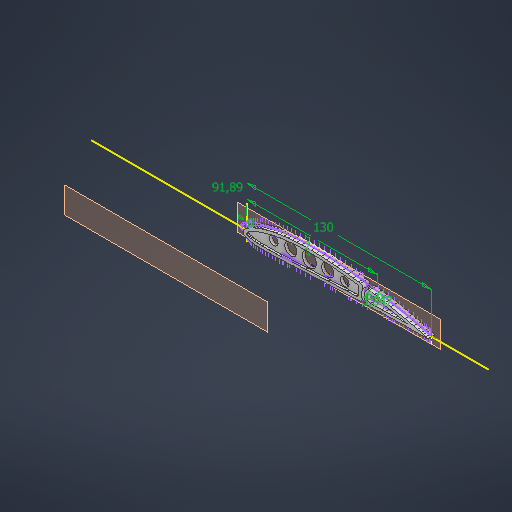
# Autodesk Inventor part: Profil NACA 4412 2
Saved by Autodesk Inventor 2026 (Build 300175050, 175E)
## iProperties
Created: 2026-02-20
Part Number: Profil NACA 4412 2
Material: Všeobecné
Document SubType Name: Modeling
Designer: marti
Density: 1 g/cm^3
Appearance: Výchozí
Author: marti
Autodesk Inventor part; units mm, degrees
ref_plane "YZ Plane" through (0, 0, 0) normal (1, 0, 0) x (0, 1, 0)
ref_plane "XZ Plane" through (0, 0, 0) normal (0, 1, 0) x (-1, 0, 0)
sketch "Náčrt1" plane through (0, 0, 0) normal (0, 0, 1) x (1, 0, 0)
  line L0 (0, 0.0009) -> (0.0949, -0.5809)
  line L1 (0.0949, -0.5809) -> (0.397, -1.1433)
  line L2 (0.397, -1.1433) -> (0.894, -1.646)
  line L3 (0.894, -1.646) -> (1.5811, -2.0907)
  line L4 (1.5811, -2.0907) -> (2.4535, -2.4793)
  line L5 (2.4535, -2.4793) -> (3.5069, -2.8138)
  line L6 (3.5069, -2.8138) -> (4.737, -3.0959)
  line L7 (4.737, -3.0959) -> (6.1391, -3.3275)
  line L8 (6.1391, -3.3275) -> (7.7086, -3.5107)
  line L9 (7.7086, -3.5107) -> (9.4408, -3.6478)
  line L10 (9.4408, -3.6478) -> (11.3308, -3.7411)
  line L11 (11.3308, -3.7411) -> (13.3737, -3.7933)
  line L12 (13.3737, -3.7933) -> (15.564, -3.7933)
  line L13 (15.564, -3.7933) -> (17.8973, -3.7933)
  line L14 (17.8973, -3.7933) -> (20.3676, -3.741)
  line L15 (20.3676, -3.741) -> (22.9712, -3.686)
  line L16 (22.9712, -3.686) -> (25.6984, -3.554)
  line L17 (25.6984, -3.554) -> (28.5465, -3.4161)
  line L18 (28.5465, -3.4161) -> (29.828, -3.3541)
  line L19 (29.828, -3.3541) -> (25.2693, -3.5754)
  line L20 (25.2693, -3.5754) -> (37.7531, -2.963)
  line L21 (37.7531, -2.963) -> (41.0259, -2.801)
  line L22 (41.0259, -2.801) -> (44.8539, -2.6115)
  line L23 (44.8539, -2.6115) -> (35.1018, -3.0226)
  line L24 (35.1018, -3.0226) -> (60.4375, -1.9699)
  line L25 (60.4375, -1.9699) -> (54.9288, -2.1938)
  line L26 (54.9288, -2.1938) -> (58.5738, -2.0455)
  line L27 (58.5738, -2.0455) -> (62.2711, -1.8951)
  line L28 (62.2711, -1.8951) -> (73.0297, -1.4573)
  line L29 (73.0297, -1.4573) -> (71.4832, -1.5215)
  line L30 (71.4832, -1.5215) -> (73.6, -1.435)
  line L31 (73.6, -1.435) -> (77.4223, -1.2826)
  line L32 (77.4223, -1.2826) -> (84.7627, -1.001)
  line L33 (87.2925, -0.9125) -> (102.9186, -0.3496)
  line L34 (102.9186, -0.3496) -> (98.1822, -0.524)
  line L35 (98.1822, -0.524) -> (96.4067, -0.572)
  line L36 (96.4067, -0.572) -> (100.0967, -0.4802)
  line L37 (100.0967, -0.4802) -> (103.7128, -0.3947)
  line L38 (103.7128, -0.3947) -> (107.2481, -0.3133)
  line L39 (107.2481, -0.3133) -> (110.6748, -0.2406)
  line L40 (110.6748, -0.2406) -> (113.9572, -0.1709)
  line L41 (113.9572, -0.1709) -> (117.1066, -0.2028)
  line L42 (117.1066, -0.2028) -> (120.0636, -0.1659)
  line L43 (120.0636, -0.1659) -> (122.7998, -0.136)
  line L44 (122.7998, -0.136) -> (127.2002, -0.0939)
  line L45 (127.2002, -0.0939) -> (127.3955, -0.0971)
  line L46 (127.3955, -0.0971) -> (129.0735, -0.125)
  line L47 (129.0735, -0.125) -> (129.9974, -0.1404)
  line L48 (129.9974, -0.1404) -> (129.9997, 0)
  line L49 (129.9997, 0) -> (128.6183, 0.5892)
  line L50 (128.6183, 0.5892) -> (126.8048, 1.0395)
  line L51 (126.8048, 1.0395) -> (125.2614, 1.446)
  line L52 (125.2614, 1.446) -> (122.7955, 2.0786)
  line L53 (122.7955, 2.0786) -> (120.0598, 2.7598)
  line L54 (120.0598, 2.7598) -> (117.1028, 3.472)
  line L55 (117.1028, 3.472) -> (113.9774, 4.2662)
  line L56 (113.9774, 4.2662) -> (110.6653, 4.9307)
  line L57 (110.6653, 4.9307) -> (107.233, 5.6192)
  line L58 (107.233, 5.6192) -> (103.7022, 6.3275)
  line L59 (103.7022, 6.3275) -> (100.087, 7.0517)
  line L60 (100.087, 7.0517) -> (96.4308, 7.7062)
  line L61 (96.4308, 7.7062) -> (92.6579, 8.3832)
  line L62 (92.6579, 8.3832) -> (87.9124, 9.1379)
  line L63 (82.4897, 9.9973) -> (81.2485, 10.1732)
  line L64 (81.2485, 10.1732) -> (77.4198, 10.673)
  line L65 (77.4198, 10.673) -> (73.598, 11.1279)
  line L66 (73.598, 11.1279) -> (69.7932, 11.5357)
  line L67 (69.7932, 11.5357) -> (66.0151, 11.8946)
  line L68 (66.0151, 11.8946) -> (62.2725, 12.2028)
  line L69 (62.2725, 12.2028) -> (58.5743, 12.4591)
  line L70 (58.5743, 12.4591) -> (54.9286, 12.6625)
  line L71 (54.9286, 12.6625) -> (51.3433, 12.8117)
  line L72 (51.3433, 12.8117) -> (47.8261, 12.889)
  line L73 (47.8261, 12.889) -> (44.3843, 12.8869)
  line L74 (44.3843, 12.8869) -> (41.025, 12.8075)
  line L75 (41.025, 12.8075) -> (37.755, 12.6532)
  line L76 (37.755, 12.6532) -> (34.5809, 12.4269)
  line L77 (34.5809, 12.4269) -> (31.509, 12.1323)
  line L78 (31.509, 12.1323) -> (28.5458, 11.773)
  line L79 (28.5458, 11.773) -> (25.6971, 11.3534)
  line L80 (25.6971, 11.3534) -> (22.969, 10.8781)
  line L81 (22.969, 10.8781) -> (20.367, 10.352)
  line L82 (20.367, 10.352) -> (17.8969, 9.7802)
  line L83 (17.8969, 9.7802) -> (15.564, 9.1684)
  line L84 (15.564, 9.1684) -> (13.3737, 8.522)
  line L85 (13.3737, 8.522) -> (11.3313, 7.8468)
  line L86 (11.3313, 7.8468) -> (9.4417, 7.1485)
  line L87 (9.4417, 7.1485) -> (7.7101, 6.433)
  line L88 (7.7101, 6.433) -> (6.1413, 5.7058)
  line L89 (6.1413, 5.7058) -> (4.74, 4.9723)
  line L90 (4.74, 4.9723) -> (3.5111, 4.2378)
  line L91 (3.5111, 4.2378) -> (2.4591, 3.5071)
  line L92 (2.4591, 3.5071) -> (1.5886, 2.7846)
  line L93 (1.5886, 2.7846) -> (0.904, 2.0741)
  line L94 (0.904, 2.0741) -> (0.4097, 1.379)
  line L95 (0.4097, 1.379) -> (0.1113, 0.7047)
  line L96 (0.1113, 0.7047) -> (0, 0.0009)
  line L97 (41.0958, 10.8086) -> (44.4086, 10.8869)
  line L98 (44.4086, 10.8869) -> (47.8048, 10.889)
  line L99 (47.8048, 10.889) -> (51.2798, 10.8126)
  line L100 (51.2798, 10.8126) -> (54.8313, 10.6648)
  line L101 (54.8313, 10.6648) -> (58.4495, 10.4629)
  line L102 (58.4495, 10.4629) -> (62.1213, 10.2085)
  line L103 (62.1213, 10.2085) -> (65.8384, 9.9023)
  line L104 (65.8384, 9.9023) -> (69.5921, 9.5458)
  line L105 (69.5921, 9.5458) -> (73.3732, 9.1405)
  line L106 (73.3732, 9.1405) -> (77.1721, 8.6884)
  line L107 (77.1721, 8.6884) -> (80.9788, 8.1915)
  line L108 (80.9788, 8.1915) -> (82.1224, 8.0294)
  line L109 (92.3241, 6.4112) -> (96.0779, 5.7375)
  line L110 (96.0779, 5.7375) -> (99.7143, 5.0866)
  line L111 (99.7143, 5.0866) -> (103.3091, 4.3665)
  line L112 (103.3091, 4.3665) -> (106.8235, 3.6615)
  line L113 (106.8235, 3.6615) -> (110.2382, 2.9765)
  line L114 (110.2382, 2.9765) -> (113.5341, 2.3153)
  line L115 (113.5341, 2.3153) -> (115.5088, 1.8135)
  line L116 (115.5088, 1.8135) -> (113.9461, 1.8293)
  line L117 (113.9461, 1.8293) -> (110.6323, 1.759)
  line L118 (110.6323, 1.759) -> (107.2038, 1.6862)
  line L119 (107.2038, 1.6862) -> (103.6661, 1.6047)
  line L120 (103.6661, 1.6047) -> (100.0482, 1.5192)
  line L121 (100.0482, 1.5192) -> (96.3548, 1.4273)
  line L122 (96.3548, 1.4273) -> (98.1184, 1.475)
  line L123 (98.1184, 1.475) -> (102.8646, 1.6498)
  line L124 (102.8646, 1.6498) -> (88.1854, 1.1209)
  line L125 (81.6875, 0.8825) -> (77.3447, 0.7159)
  line L126 (77.3447, 0.7159) -> (73.5193, 0.5634)
  line L127 (73.5193, 0.5634) -> (71.4009, 0.4768)
  line L128 (71.4009, 0.4768) -> (72.9476, 0.541)
  line L129 (72.9476, 0.541) -> (62.1898, 0.1033)
  line L130 (62.1898, 0.1033) -> (58.4925, -0.0472)
  line L131 (58.4925, -0.0472) -> (54.8476, -0.1955)
  line L132 (54.8476, -0.1955) -> (60.3554, 0.0284)
  line L133 (60.3554, 0.0284) -> (35.0182, -1.0243)
  line L134 (35.0182, -1.0243) -> (44.7624, -0.6136)
  line L135 (44.7624, -0.6136) -> (40.9263, -0.8035)
  line L136 (40.9263, -0.8035) -> (37.6546, -0.9654)
  line L137 (37.6546, -0.9654) -> (25.1718, -1.5778)
  line L138 (25.1718, -1.5778) -> (29.7312, -1.3564)
  line L139 (29.7312, -1.3564) -> (28.4563, -1.4181)
  line L140 (28.4563, -1.4181) -> (25.6082, -1.556)
  line L141 (25.6082, -1.556) -> (22.9017, -1.687)
  line L142 (22.9017, -1.687) -> (20.3188, -1.7416)
  line L143 (20.3188, -1.7416) -> (17.8761, -1.7933)
  line L144 (17.8761, -1.7933) -> (15.564, -1.7933)
  line L145 (15.564, -1.7933) -> (13.3992, -1.7933)
  line L146 (13.3992, -1.7933) -> (11.4056, -1.7424)
  line L147 (11.4056, -1.7424) -> (9.569, -1.6517)
  line L148 (9.569, -1.6517) -> (7.9035, -1.5199)
  line L149 (7.9035, -1.5199) -> (6.4182, -1.3465)
  line L150 (6.4182, -1.3465) -> (5.1239, -1.1327)
  line L151 (5.1239, -1.1327) -> (4.034, -0.8827)
  line L152 (4.034, -0.8827) -> (3.1652, -0.6069)
  line L153 (3.1652, -0.6069) -> (2.5371, -0.3271)
  line L154 (2.5371, -0.3271) -> (2.1633, -0.0851)
  line L155 (2.1633, -0.0851) -> (2.0322, 0.0474)
  line L156 (2.0322, 0.0474) -> (2.046, 0.1343)
  line L157 (2.046, 0.1343) -> (2.1568, 0.3847)
  line L158 (2.1568, 0.3847) -> (2.4476, 0.7937)
  line L159 (2.4476, 0.7937) -> (2.9515, 1.3167)
  line L160 (2.9515, 1.3167) -> (3.6705, 1.9134)
  line L161 (3.6705, 1.9134) -> (4.5959, 2.5562)
  line L162 (4.5959, 2.5562) -> (5.7176, 3.2266)
  line L163 (5.7176, 3.2266) -> (7.0261, 3.9115)
  line L164 (7.0261, 3.9115) -> (8.5129, 4.6007)
  line L165 (8.5129, 4.6007) -> (10.1705, 5.2857)
  line L166 (10.1705, 5.2857) -> (11.992, 5.9587)
  line L167 (11.992, 5.9587) -> (13.9708, 6.6129)
  line L168 (13.9708, 6.6129) -> (16.1009, 7.2416)
  line L169 (16.1009, 7.2416) -> (18.3762, 7.8383)
  line L170 (18.3762, 7.8383) -> (20.7908, 8.3972)
  line L171 (20.7908, 8.3972) -> (23.3389, 8.9124)
  line L172 (23.3389, 8.9124) -> (26.0146, 9.3786)
  line L173 (26.0146, 9.3786) -> (28.8119, 9.7907)
  line L174 (28.8119, 9.7907) -> (31.7249, 10.1438)
  line L175 (31.7249, 10.1438) -> (34.7474, 10.4337)
  line L176 (34.7474, 10.4337) -> (37.8732, 10.6565)
  line L177 (37.8732, 10.6565) -> (41.0958, 10.8086)
  line L178 (0, 16.2255) -> (0, -7.1297) projected
  line L179 (-109.522, 0) -> (169.92, 0) projected
  arc A0 (85.4115, 9.5353) -> (84.7627, -1.001) centre (91.8618, 3.85) ccw
  arc A1 (87.9203, 9.1438) -> (87.2925, -0.9125) centre (91.8618, 3.85) ccw
  line L180 (85.4115, 9.5353) -> (82.4897, 9.9973)
  arc A2 (92.7028, 8.3752) -> (92.6128, 8.3904) centre (91.8903, 3.8474) ccw
  line L181 (88.551, 7.0112) -> (92.3241, 6.4112)
  arc A3 (82.1224, 8.0294) -> (81.6875, 0.8825) centre (91.8618, 3.85) ccw
  arc A4 (88.551, 7.0112) -> (88.1854, 1.1209) centre (91.8903, 3.8474) ccw
  point P0 (0, 0)
  point P1 (0.0092, 0.0443)
  point P2 (80.0237, 10.3925)
  point P3 (81.2485, -1.1461)
  point P4 (85.0783, -0.9923)
  point P5 (0, -1.8302)
  point P6 (0, -1.8314)
  point P7 (72.2186, -1.4898)
  point P8 (-4.2032, 0)
  point P9 (0, 0.1702)
  point P10 (129.7617, -0.163)
  point P11 (0, 11.0071)
  point P12 (0, -1.8299)
  point P13 (41.3587, -2.7449)
  point P14 (41.277, -0.7466)
  point P15 (0, 8.9957)
  point P16 (0, 0.1718)
  point P17 (0, 0.1714)
  point P18 (-69.6017, 0)
  point P19 (72.1378, 0.5085)
  point P20 (26.1583, -1.5294)
  point P21 (59.6518, 0)
  point P22 (2.0791, 0)
  point P23 (26.2556, -3.527)
  point P24 (44.1123, -2.6482)
  point P25 (44.0214, -0.6503)
  point P26 (59.6564, 0)
  point P27 (97.4348, 1.4542)
  point P28 (97.4969, -0.5449)
  point P29 (97.7601, -0.5354)
  point P30 (87.9124, 9.1379)
  point P31 (97.6955, 1.4636)
  point P32 (59.6716, 0)
  dimension "d0" = 2
  dimension "d1" = 0
  dimension "d10" = 129.9997
  dimension "d12" = 3.8474
  dimension "d13" = 91.8903
  dimension "d17" = 6.6
  constraints: 360 end point, 12 collinear, 11 point on circle, 5 centre point, 3 coincident, 3 point on line, 2 parallel, 2 perpendicular, 2 tangent, 1 horizontal, 75 other
  measures "d0" distance between parallel lines of L74 L97
  measures "d1" distance from line of L178 point (0, 0.001)
  measures "d10" distance of L48.end point (0, 0.001)
  measures "d12" distance from line of L179 A2.centre
  measures "d13" distance from line of L178 A2.centre
  measures "d17" radius of A1
ref_plane "Pracovní rovina1" through (0, 0, 50) normal (0, 0, 1) x (1, 0, 0)
sketch "Náčrt2" plane through (0.1197, -0.0139, 50) normal (0, 0, 1) x (1, 0, 0)
  line L0 (-71.7303, -0.321) -> (-71.6354, -0.9019)
  line L1 (-71.6354, -0.9019) -> (-71.3333, -1.4643)
  line L2 (-71.3333, -1.4643) -> (-70.8362, -1.967)
  line L3 (-70.8362, -1.967) -> (-70.1492, -2.4117)
  line L4 (-70.1492, -2.4117) -> (-69.2768, -2.8003)
  line L5 (-69.2768, -2.8003) -> (-68.2233, -3.1347)
  line L6 (-68.2233, -3.1347) -> (-66.9933, -3.4168)
  line L7 (-66.9933, -3.4168) -> (-65.5912, -3.6485)
  line L8 (-65.5912, -3.6485) -> (-64.0217, -3.8317)
  line L9 (-64.0217, -3.8317) -> (-62.2895, -3.9688)
  line L10 (-62.2895, -3.9688) -> (-60.3995, -4.0621)
  line L11 (-60.3995, -4.0621) -> (-58.3565, -4.1142)
  line L12 (-58.3565, -4.1142) -> (-56.1662, -4.1142)
  line L13 (-56.1662, -4.1142) -> (-53.833, -4.1142)
  line L14 (-53.833, -4.1142) -> (-51.3627, -4.062)
  line L15 (-51.3627, -4.062) -> (-48.7592, -4.0069)
  line L16 (-48.7592, -4.0069) -> (-46.0319, -3.8749)
  line L17 (-46.0319, -3.8749) -> (-43.1838, -3.7371)
  line L18 (-43.1838, -3.7371) -> (-40.2179, -3.5936)
  line L19 (-40.2179, -3.5936) -> (-37.15, -3.4367)
  line L20 (-37.15, -3.4367) -> (-33.9745, -3.2772)
  line L21 (-33.9745, -3.2772) -> (-30.7049, -3.1104)
  line L22 (-30.7049, -3.1104) -> (-27.346, -2.9391)
  line L23 (-27.346, -2.9391) -> (-23.9054, -2.7954)
  line L24 (-23.9054, -2.7954) -> (-23.4055, -2.7752)
  line L25 (-23.4055, -2.7752) -> (-16.802, -2.5148)
  line L26 (-16.802, -2.5148) -> (-13.1565, -2.3665)
  line L27 (-13.1565, -2.3665) -> (-9.459, -2.216)
  line L28 (-9.459, -2.216) -> (1.2996, -1.7761)
  line L29 (1.2996, -1.7761) -> (-1.939, -1.9065)
  line L30 (-1.939, -1.9065) -> (1.8675, -1.757)
  line L31 (1.8675, -1.757) -> (5.6913, -1.6068)
  line L32 (5.6913, -1.6068) -> (13.346, -1.3203)
  line L33 (13.346, -1.3203) -> (17.1555, -1.1884)
  line L34 (17.1555, -1.1884) -> (20.9379, -1.0676)
  line L35 (20.9379, -1.0676) -> (24.6804, -0.9571)
  line L36 (24.6804, -0.9571) -> (28.3686, -0.8572)
  line L37 (28.3686, -0.8572) -> (31.9862, -0.7683)
  line L38 (31.9862, -0.7683) -> (35.5166, -0.6903)
  line L39 (35.5166, -0.6903) -> (38.9405, -0.6229)
  line L40 (38.9405, -0.6229) -> (42.2338, -0.5655)
  line L41 (42.2338, -0.5655) -> (45.3763, -0.5685)
  line L42 (45.3763, -0.5685) -> (48.3339, -0.5316)
  line L43 (48.3339, -0.5316) -> (51.07, -0.5017)
  line L44 (51.07, -0.5017) -> (53.5363, -0.4781)
  line L45 (53.5363, -0.4781) -> (55.6645, -0.46)
  line L46 (55.6645, -0.46) -> (57.343, -0.4458)
  line L47 (57.343, -0.4458) -> (58.272, -0.4379)
  line L48 (58.272, -0.4379) -> (58.2695, -0.1446)
  line L49 (58.2695, -0.1446) -> (57.3365, 0.1109)
  line L50 (57.3365, 0.1109) -> (55.6584, 0.5623)
  line L51 (55.6584, 0.5623) -> (53.5305, 1.1227)
  line L52 (53.5305, 1.1227) -> (51.0647, 1.7553)
  line L53 (51.0647, 1.7553) -> (48.329, 2.4365)
  line L54 (48.329, 2.4365) -> (45.372, 3.1487)
  line L55 (45.372, 3.1487) -> (42.2483, 3.9465)
  line L56 (42.2483, 3.9465) -> (38.9352, 4.6104)
  line L57 (38.9352, 4.6104) -> (35.5028, 5.2982)
  line L58 (35.5028, 5.2982) -> (31.9708, 6.006)
  line L59 (31.9708, 6.006) -> (28.356, 6.7272)
  line L60 (28.356, 6.7272) -> (24.6665, 7.3905)
  line L61 (24.6665, 7.3905) -> (20.9275, 8.0618)
  line L62 (20.9275, 8.0618) -> (17.1433, 8.6633)
  line L63 (17.1433, 8.6633) -> (10.7595, 9.6764)
  line L64 (10.7595, 9.6764) -> (9.5183, 9.8523)
  line L65 (9.5183, 9.8523) -> (5.6895, 10.352)
  line L66 (5.6895, 10.352) -> (1.8677, 10.8069)
  line L67 (1.8677, 10.8069) -> (-1.937, 11.2148)
  line L68 (-1.937, 11.2148) -> (-5.7152, 11.5736)
  line L69 (-5.7152, 11.5736) -> (-9.4577, 11.8818)
  line L70 (-9.4577, 11.8818) -> (-13.156, 12.1381)
  line L71 (-13.156, 12.1381) -> (-16.8017, 12.3415)
  line L72 (-16.8017, 12.3415) -> (-20.3869, 12.4907)
  line L73 (-20.3869, 12.4907) -> (-23.9041, 12.568)
  line L74 (-23.9041, 12.568) -> (-27.3459, 12.5659)
  line L75 (-27.3459, 12.5659) -> (-30.7053, 12.4865)
  line L76 (-30.7053, 12.4865) -> (-33.9753, 12.3322)
  line L77 (-33.9753, 12.3322) -> (-37.1494, 12.106)
  line L78 (-37.1494, 12.106) -> (-40.2212, 11.8113)
  line L79 (-40.2212, 11.8113) -> (-43.1845, 11.4521)
  line L80 (-43.1845, 11.4521) -> (-46.0331, 11.0325)
  line L81 (-46.0331, 11.0325) -> (-48.7613, 10.5571)
  line L82 (-48.7613, 10.5571) -> (-51.3633, 10.031)
  line L83 (-51.3633, 10.031) -> (-53.8334, 9.4593)
  line L84 (-53.8334, 9.4593) -> (-56.1663, 8.8474)
  line L85 (-56.1663, 8.8474) -> (-58.3565, 8.201)
  line L86 (-58.3565, 8.201) -> (-60.399, 7.5258)
  line L87 (-60.399, 7.5258) -> (-62.2885, 6.8276)
  line L88 (-62.2885, 6.8276) -> (-64.0202, 6.112)
  line L89 (-64.0202, 6.112) -> (-65.589, 5.3848)
  line L90 (-65.589, 5.3848) -> (-66.9902, 4.6513)
  line L91 (-66.9902, 4.6513) -> (-68.2191, 3.9168)
  line L92 (-68.2191, 3.9168) -> (-69.2711, 3.1861)
  line L93 (-69.2711, 3.1861) -> (-70.1417, 2.4636)
  line L94 (-70.1417, 2.4636) -> (-70.8263, 1.7531)
  line L95 (-70.8263, 1.7531) -> (-71.3206, 1.058)
  line L96 (-71.3206, 1.058) -> (-71.6181, 0.3856)
  line L97 (-71.6181, 0.3856) -> (-71.7303, -0.321)
  line L98 (-30.6345, 10.4876) -> (-27.3217, 10.566)
  line L99 (-27.3217, 10.566) -> (-23.9255, 10.568)
  line L100 (-23.9255, 10.568) -> (-20.4505, 10.4916)
  line L101 (-20.4505, 10.4916) -> (-16.899, 10.3438)
  line L102 (-16.899, 10.3438) -> (-13.2808, 10.142)
  line L103 (-13.2808, 10.142) -> (-9.6089, 9.8875)
  line L104 (-9.6089, 9.8875) -> (-5.8918, 9.5814)
  line L105 (-5.8918, 9.5814) -> (-2.1382, 9.2249)
  line L106 (-2.1382, 9.2249) -> (1.6429, 8.8196)
  line L107 (1.6429, 8.8196) -> (5.4419, 8.3674)
  line L108 (5.4419, 8.3674) -> (9.2485, 7.8705)
  line L109 (9.2485, 7.8705) -> (10.4624, 7.6985)
  line L110 (10.4624, 7.6985) -> (16.8296, 6.6881)
  line L111 (16.8296, 6.6881) -> (20.5938, 6.0898)
  line L112 (20.5938, 6.0898) -> (24.3128, 5.422)
  line L113 (24.3128, 5.422) -> (27.9834, 4.7621)
  line L114 (27.9834, 4.7621) -> (31.5786, 4.0448)
  line L115 (31.5786, 4.0448) -> (35.0933, 3.3405)
  line L116 (35.0933, 3.3405) -> (38.508, 2.6563)
  line L117 (38.508, 2.6563) -> (41.8041, 1.9958)
  line L118 (41.8041, 1.9958) -> (44.0083, 1.4328)
  line L119 (44.0083, 1.4328) -> (42.2173, 1.4345)
  line L120 (42.2173, 1.4345) -> (38.9034, 1.3767)
  line L121 (38.9034, 1.3767) -> (35.4748, 1.3092)
  line L122 (35.4748, 1.3092) -> (31.9395, 1.2311)
  line L123 (31.9395, 1.2311) -> (28.3169, 1.1421)
  line L124 (28.3169, 1.1421) -> (24.6238, 1.0421)
  line L125 (24.6238, 1.0421) -> (20.8764, 0.9314)
  line L126 (20.8764, 0.9314) -> (17.089, 0.8105)
  line L127 (17.089, 0.8105) -> (13.274, 0.6784)
  line L128 (13.274, 0.6784) -> (5.6146, 0.3917)
  line L129 (5.6146, 0.3917) -> (1.789, 0.2415)
  line L130 (1.789, 0.2415) -> (-2.0185, 0.0919)
  line L131 (-2.0185, 0.0919) -> (1.2185, 0.2222)
  line L132 (1.2185, 0.2222) -> (-9.5405, -0.2177)
  line L133 (-9.5405, -0.2177) -> (-13.2378, -0.3681)
  line L134 (-13.2378, -0.3681) -> (-16.8821, -0.5164)
  line L135 (-16.8821, -0.5164) -> (-23.4852, -0.7768)
  line L136 (-23.4852, -0.7768) -> (-23.9874, -0.797)
  line L137 (-23.9874, -0.797) -> (-27.4387, -0.9412)
  line L138 (-27.4387, -0.9412) -> (-30.8046, -1.1129)
  line L139 (-30.8046, -1.1129) -> (-34.0757, -1.2797)
  line L140 (-34.0757, -1.2797) -> (-37.2512, -1.4393)
  line L141 (-37.2512, -1.4393) -> (-40.3173, -1.596)
  line L142 (-40.3173, -1.596) -> (-43.274, -1.7391)
  line L143 (-43.274, -1.7391) -> (-46.122, -1.877)
  line L144 (-46.122, -1.877) -> (-48.8287, -2.008)
  line L145 (-48.8287, -2.008) -> (-51.4115, -2.0626)
  line L146 (-51.4115, -2.0626) -> (-53.8541, -2.1142)
  line L147 (-53.8541, -2.1142) -> (-56.1662, -2.1142)
  line L148 (-56.1662, -2.1142) -> (-58.331, -2.1142)
  line L149 (-58.331, -2.1142) -> (-60.3246, -2.0633)
  line L150 (-60.3246, -2.0633) -> (-62.1613, -1.9727)
  line L151 (-62.1613, -1.9727) -> (-63.8267, -1.8409)
  line L152 (-63.8267, -1.8409) -> (-65.3121, -1.6675)
  line L153 (-65.3121, -1.6675) -> (-66.6064, -1.4537)
  line L154 (-66.6064, -1.4537) -> (-67.6963, -1.2037)
  line L155 (-67.6963, -1.2037) -> (-68.565, -0.9279)
  line L156 (-68.565, -0.9279) -> (-69.1931, -0.6481)
  line L157 (-69.1931, -0.6481) -> (-69.5669, -0.4061)
  line L158 (-69.5669, -0.4061) -> (-69.6978, -0.2738)
  line L159 (-69.6978, -0.2738) -> (-69.6837, -0.1853)
  line L160 (-69.6837, -0.1853) -> (-69.5735, 0.0638)
  line L161 (-69.5735, 0.0638) -> (-69.2827, 0.4727)
  line L162 (-69.2827, 0.4727) -> (-68.7787, 0.9957)
  line L163 (-68.7787, 0.9957) -> (-68.0598, 1.5924)
  line L164 (-68.0598, 1.5924) -> (-67.1344, 2.2352)
  line L165 (-67.1344, 2.2352) -> (-66.0127, 2.9056)
  line L166 (-66.0127, 2.9056) -> (-64.7042, 3.5905)
  line L167 (-64.7042, 3.5905) -> (-63.2174, 4.2797)
  line L168 (-63.2174, 4.2797) -> (-61.5597, 4.9647)
  line L169 (-61.5597, 4.9647) -> (-59.7383, 5.6378)
  line L170 (-59.7383, 5.6378) -> (-57.7594, 6.292)
  line L171 (-57.7594, 6.292) -> (-55.6294, 6.9206)
  line L172 (-55.6294, 6.9206) -> (-53.3541, 7.5173)
  line L173 (-53.3541, 7.5173) -> (-50.9395, 8.0762)
  line L174 (-50.9395, 8.0762) -> (-48.3914, 8.5915)
  line L175 (-48.3914, 8.5915) -> (-45.7157, 9.0576)
  line L176 (-45.7157, 9.0576) -> (-42.9184, 9.4697)
  line L177 (-42.9184, 9.4697) -> (-40.0053, 9.8229)
  line L178 (-40.0053, 9.8229) -> (-36.9828, 10.1128)
  line L179 (-36.9828, 10.1128) -> (-33.857, 10.3355)
  line L180 (-33.857, 10.3355) -> (-30.6345, 10.4876)
  line L181 (0, 15.9045) -> (0, -7.4507)
  line L182 (-97.7307, 0) -> (84.2724, 0)
  point P0 (0, 0)
  point P1 (-71.7211, -0.2767)
  point P2 (9.5183, -1.467)
  point P3 (0, -1.8293)
  point P4 (0, -1.8303)
  point P5 (-0.6652, -1.8565)
  point P6 (-4.2164, 0)
  point P7 (0, 0.1712)
  dimension "d6" = 2
  dimension "d5" = 71.7303
  constraints: 366 end point, 12 collinear, 3 perpendicular, 2 parallel, 1 coincident, 1 horizontal, 82 other
  measures "d6" distance between parallel lines of L75 L98
  measures "d5" distance from line of L181 point (-71.73, -0.321)
extrude "Vysunutí2" [suppressed]
ref_plane "Pracovní rovina3" through (0, 0, 0) normal (0, 0, 1) x (1, 0, 0)
sketch "Náčrt3" plane through (0, 0, 0) normal (0, 0, 1) x (1, 0, 0)
  arc A0 (83.961, 7.2422) -> (82.4897, 9.9973) centre (82.1232, 8.0312) ccw projected
  line L0 (82.4897, 9.9973) -> (81.2485, 10.1732) projected
  line L1 (81.2485, 10.1732) -> (77.4198, 10.673) projected
  line L2 (77.4198, 10.673) -> (73.598, 11.1279) projected
  line L3 (73.598, 11.1279) -> (69.7932, 11.5357) projected
  line L4 (69.7932, 11.5357) -> (66.0151, 11.8946) projected
  line L5 (66.0151, 11.8946) -> (62.2725, 12.2028) projected
  line L6 (62.2725, 12.2028) -> (58.5743, 12.4591) projected
  line L7 (58.5743, 12.4591) -> (54.9286, 12.6625) projected
  line L8 (54.9286, 12.6625) -> (51.3433, 12.8117) projected
  line L9 (51.3433, 12.8117) -> (47.8261, 12.889) projected
  line L10 (47.8261, 12.889) -> (44.3843, 12.8869) projected
  line L11 (44.3843, 12.8869) -> (41.025, 12.8075) projected
  line L12 (41.025, 12.8075) -> (37.755, 12.6532) projected
  line L13 (37.755, 12.6532) -> (34.5809, 12.4269) projected
  line L14 (34.5809, 12.4269) -> (31.509, 12.1323) projected
  line L15 (31.509, 12.1323) -> (28.5458, 11.773) projected
  line L16 (28.5458, 11.773) -> (25.6971, 11.3534) projected
  line L17 (25.6971, 11.3534) -> (22.969, 10.8781) projected
  line L18 (22.969, 10.8781) -> (20.367, 10.352) projected
  line L19 (20.367, 10.352) -> (17.8969, 9.7802) projected
  line L20 (17.8969, 9.7802) -> (15.564, 9.1684) projected
  line L21 (15.564, 9.1684) -> (13.3737, 8.522) projected
  line L22 (13.3737, 8.522) -> (11.3313, 7.8468) projected
  line L23 (11.3313, 7.8468) -> (9.4417, 7.1485) projected
  line L24 (9.4417, 7.1485) -> (7.7101, 6.433) projected
  line L25 (7.7101, 6.433) -> (6.1413, 5.7058) projected
  line L26 (6.1413, 5.7058) -> (4.74, 4.9723) projected
  line L27 (4.74, 4.9723) -> (3.5111, 4.2378) projected
  line L28 (3.5111, 4.2378) -> (2.4591, 3.5071) projected
  line L29 (2.4591, 3.5071) -> (1.5886, 2.7846) projected
  line L30 (1.5886, 2.7846) -> (0.904, 2.0741) projected
  line L31 (0.904, 2.0741) -> (0.4097, 1.379) projected
  line L32 (0.4097, 1.379) -> (0.1113, 0.7047) projected
  line L33 (0.1113, 0.7047) -> (0, 0.0009) projected
  line L34 (0, 0.0009) -> (0.0949, -0.5809) projected
  line L35 (0.0949, -0.5809) -> (0.397, -1.1433) projected
  line L36 (0.397, -1.1433) -> (0.894, -1.646) projected
  line L37 (0.894, -1.646) -> (1.5811, -2.0907) projected
  line L38 (1.5811, -2.0907) -> (2.4535, -2.4793) projected
  line L39 (2.4535, -2.4793) -> (3.5069, -2.8138) projected
  line L40 (3.5069, -2.8138) -> (4.737, -3.0959) projected
  line L41 (4.737, -3.0959) -> (6.1391, -3.3275) projected
  line L42 (6.1391, -3.3275) -> (7.7086, -3.5107) projected
  line L43 (7.7086, -3.5107) -> (9.4408, -3.6478) projected
  line L44 (9.4408, -3.6478) -> (11.3308, -3.7411) projected
  line L45 (11.3308, -3.7411) -> (13.3737, -3.7933) projected
  line L46 (13.3737, -3.7933) -> (17.8973, -3.7933) projected
  line L47 (17.8973, -3.7933) -> (22.9712, -3.686) projected
  line L48 (22.9712, -3.686) -> (26.2556, -3.527) projected
  line L49 (26.2556, -3.527) -> (37.7531, -2.963) projected
  line L50 (37.7531, -2.963) -> (44.1123, -2.6482) projected
  line L51 (44.1123, -2.6482) -> (35.1018, -3.0226) projected
  line L52 (35.1018, -3.0226) -> (44.8539, -2.6115) projected
  line L53 (44.8539, -2.6115) -> (44.1123, -2.6482) projected
  line L54 (44.1123, -2.6482) -> (60.4375, -1.9699) projected
  line L55 (60.4375, -1.9699) -> (54.9288, -2.1938) projected
  line L56 (54.9288, -2.1938) -> (62.2711, -1.8951) projected
  line L57 (62.2711, -1.8951) -> (73.0297, -1.4573) projected
  line L58 (73.0297, -1.4573) -> (71.4832, -1.5215) projected
  line L59 (71.4832, -1.5215) -> (73.6, -1.435) projected
  line L60 (73.6, -1.435) -> (77.4223, -1.2826) projected
  line L61 (77.4223, -1.2826) -> (81.7641, -1.116) projected
  arc A1 (81.7641, -1.116) -> (83.6075, 1.4425) centre (81.6875, 0.8825) ccw projected
  arc A2 (83.961, 7.2422) -> (83.6075, 1.4425) centre (91.8618, 3.85) ccw projected
  line L62 (-5.5732, 4) -> (145.5295, 4) construction
  line L63 (-35.7938, 0) -> (175.7501, 0) projected
  line L64 (0, 16.2255) -> (0, -7.1297) projected
  circle A3 centre (20, 4) radius 3
  circle A4 centre (70, 4) radius 3
  line L65 (0, 5) -> (133.2709, 5) construction
  circle A5 centre (45, 5) radius 5
  circle A6 centre (32, 5) radius 4.25
  circle A7 centre (58, 5) radius 4.25
  point P0 (0, 0)
  point P1 (59.6518, 0)
  point P2 (59.6564, 0)
  dimension "d31" = 6
  dimension "d32" = 6
  dimension "d33" = 20
  dimension "d34" = 70
  dimension "d37" = 5
  dimension "d39" = 10
  dimension "d40" = 8.5
  dimension "d41" = 8.5
  dimension "d42" = 45
  dimension "d43" = 32
  dimension "d44" = 58
  constraints: 5 centre point, 4 end point, 4 point on line, 2 horizontal, 2 other
  measures "d31" diameter of A3
  measures "d32" diameter of A4
  measures "d37" distance between parallel lines of L63 L65
  measures "d39" diameter of A5
  measures "d40" diameter of A6
  measures "d41" diameter of A7
extrude "Vysunutí7" add sketch "Náčrt1" along normal mid plane 5 contours L179 L155 L154 L153 L152 L151 L150 L149 L148 L147 L146 L145 L144 L143 L142 L141 L137 L136 L135 L133 L130 A0 L32 L31 L30 L28 L27 L24 L22 L21 L20 L17 L16 L15 L14 L13 L12 L11 L10 L9 L8 L7 L6 L5 L4 L3 L2 L1 L0 | L96 L95 L94 L93 L92 L91 L90 L89 L88 L87 L86 L85 L84 L83 L82 L81 L80 L79 L78 L77 L76 L75 L74 L73 L72 L71 L70 L69 L68 L67 L66 L65 L64 L63 L180 A0 L179 L130 L129 L127 L126 L125 A3 L108 L107 L106 L105 L104 L103 L102 L101 L100 L99 L98 L97 L177 L176 L175 L174 L173 L172 L171 L170 L169 L168 L167 L166 L165 L164 L163 L162 L161 L160 L159 L158 L157 L156 L155
extrude "Vysunutí8" add sketch "Náčrt1" along normal mid plane 5 contours A1 L62 L61 L60 L59 L58 L57 L56 L55 L54 L53 L52 L51 L50 L49 L179 | L179 L48 L47 L46 L45 L44 L43 L42 L41 L40 L39 L38 L37 L36 L33 A1
extrude "Vysunutí9" add sketch "Náčrt3" along normal mid plane 2
fillet "Zaoblení6" radius 2 10 edges at (85.4115, 9.5353, 1.25) (85.4115, 9.5353, -1.25) (84.7627, -1.001, 1.25) (84.7627, -1.001, -1.25) (81.6875, 0.8825, 1.75) (81.6875, 0.8825, -1.75) (82.1224, 8.0294, -1.75) (82.1224, 8.0294, 1.75) (80.9788, 8.1915, 1.75) (80.9788, 8.1915, -1.75)
fillet "Zaoblení7" radius 2 4 edges at (88.551, 7.0112, 0) (88.1854, 1.1209, 0) (87.2925, -0.9125, 0) (87.9124, 9.1379, 0)
